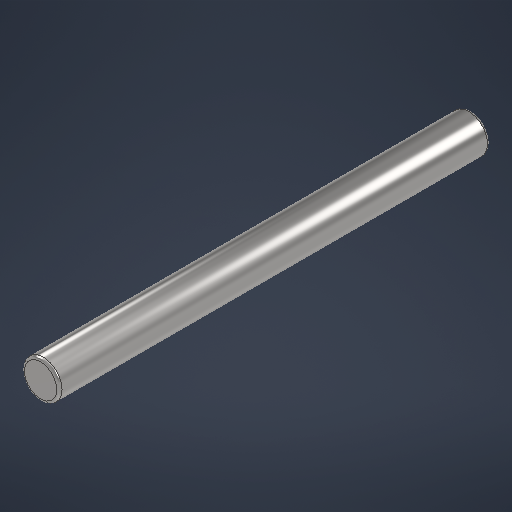
# Autodesk Inventor part: HIN-61 BISAGRA (PASADOR)
Saved by Autodesk Inventor 2025 (Build 290162000, 162)
## iProperties
Created: 2026-02-04
Part Number: HIN-61 BISAGRA (PASADOR)
Material: Acero inoxidable
Document SubType Name: Modeling
Designer: ROLANDO
Density: 8 g/cm^3
Appearance: Semipulido
Author: ROLANDO
Autodesk Inventor part; units mm, degrees
ref_plane "YZ Plane" through (0, 0, 0) normal (1, 0, 0) x (0, 1, 0)
ref_plane "XZ Plane" through (0, 0, 0) normal (0, 1, 0) x (-1, 0, 0)
ref_plane "XY Plane" through (0, 0, 0) normal (0, 0, 1) x (1, 0, 0)
sketch "Boceto1" plane through (0, 0, 0) normal (0, 0, 1) x (1, 0, 0)
  circle A0 centre (0, 0) radius 3.5
  dimension "d0" = 7
  constraints: 1 centre point, 1 coincident
  measures "d0" diameter of A0
extrude "Extrusión1" add sketch "Boceto1" against normal blind 80
fillet "Empalme1" radius 0.5 2 edges at (-3.5, 0, 0) (-3.5, 0, -80)
